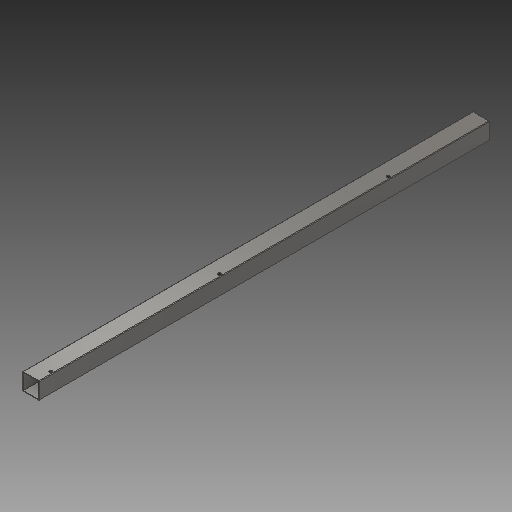
# Autodesk Inventor part: TABLE_BERAM
Saved by Autodesk Inventor 2019 (Build 230136000, 136)
## iProperties
Created: 2019-02-24
Part Number: TABLE_BERAM
Material: Stainless Steel
Document SubType Name: Modeling
Designer: gaincarlo
Density: 8 g/cm^3
Appearance: Semi-Polished
Author: gaincarlo
Autodesk Inventor part; units mm, degrees
ref_plane "YZ Plane" through (0, 0, 0) normal (1, 0, 0) x (0, 1, 0)
ref_plane "XZ Plane" through (0, 0, 0) normal (0, 1, 0) x (-1, 0, 0)
ref_plane "XY Plane" through (0, 0, 0) normal (0, 0, 1) x (1, 0, 0)
sketch "Sketch1" plane through (0, 0, 0) normal (0, 0, 1) x (1, 0, 0)
  line L0 (-28, 30) -> (28, 30)
  line L1 (30, 28) -> (30, -28)
  line L2 (28, -30) -> (-28, -30)
  line L3 (-30, -28) -> (-30, 28)
  line L4 (-30, 30) -> (30, -30) construction
  line L5 (28, 28) -> (-28, 28)
  line L6 (-28, 28) -> (-28, -28)
  line L7 (-28, -28) -> (28, -28)
  line L8 (28, -28) -> (28, 28)
  arc A0 (-28, 30) -> (-30, 28) centre (-28, 28) ccw
  arc A1 (30, 28) -> (28, 30) centre (28, 28) ccw
  arc A2 (28, -30) -> (30, -28) centre (28, -28) ccw
  arc A3 (-30, -28) -> (-28, -30) centre (-28, -28) ccw
  point P0 (0, 0)
  point P1 (30, 30)
  point P2 (-30, -30)
  point P3 (0, 0)
  dimension "d0" = 60
  dimension "d1" = 60
  dimension "d2" = 2
  dimension "d3" = 2
  constraints: 18 end point, 8 point on circle, 8 point on line, 8 tangent, 4 centre point, 4 parallel, 3 equal radius, 2 perpendicular, 1 coincident, 1 horizontal, 1 midpoint, 3 other
  measures "d0" distance of L4.end point (-30, -30)
  measures "d1" distance of point (30, 30) L4.end
  measures "d2" distance between parallel lines of L0 L5
  measures "d3" radius of A0
extrude "Extrusion1" add sketch "Sketch1" along normal blind 1600
sketch "Sketch2" plane through (-28, 30, 0) normal (0, 1, 0) x (1, 0, 0)
  circle A0 centre (48, -950) radius 5
  line L0 (56, -1600) -> (0, -1600) projected
  line L1 (56, 0) -> (0, 0) projected
  circle A1 centre (48, -350) radius 5
  circle A2 centre (48, -1550) radius 5
  line L2 (48, -116) -> (48, -1518) construction
  line L3 (58, 0) -> (58, -1600) projected
  point P0 (28, 0)
  dimension "d6" = 10
  dimension "d10" = 950
  dimension "d11" = 10
  dimension "d12" = 10
  dimension "d13" = 600
  dimension "d14" = 600
  dimension "d15" = 10
  constraints: 3 centre point, 3 point on line, 2 end point, 1 vertical
  measures "d6" diameter of A0
  measures "d10" distance from line of L1 A0.centre
  measures "d11" diameter of A1
  measures "d12" diameter of A2
  measures "d13" distance of A0.centre A1.centre
  measures "d14" distance of A2.centre A0.centre
  measures "d15" distance between parallel lines of L3 L2
extrude "Extrusion2" cut sketch "Sketch2" against normal up to next
body "Solid1"
